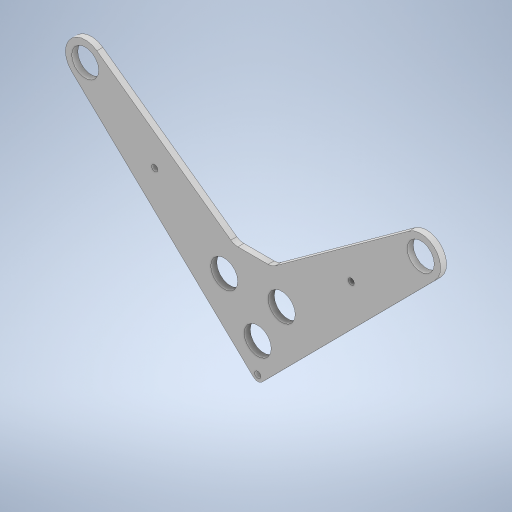
# Autodesk Inventor part: MainBody
Saved by Autodesk Inventor 2024.3 (Build 283343000, 343)
## iProperties
Created: 2024-09-01
Part Number: MainBody
Material: Generic
Document SubType Name: Modeling
Designer: isaac
Density: 1 g/cm^3
Appearance: Default
Author: isaac
Autodesk Inventor part; units mm, degrees
ref_plane "YZ Plane" through (0, 0, 0) normal (1, 0, 0) x (0, 1, 0)
ref_plane "XZ Plane" through (0, 0, 0) normal (0, 1, 0) x (-1, 0, 0)
ref_plane "XY Plane" through (0, 0, 0) normal (0, 0, 1) x (1, 0, 0)
sketch "Sketch1" plane through (0, 0, 0) normal (0, 0, 1) x (1, 0, 0)
  circle A0 centre (0, 0) radius 20.32 construction
  circle A1 centre (25.4496, 43.9654) radius 30.48 construction
  circle A2 centre (-35.5104, 43.9654) radius 30.48 construction
  circle A3 centre (-35.5104, 43.9654) radius 31.75 construction
  circle A4 centre (0, 0) radius 21.59 construction
  line L0 (-15.5607, 19.2657) -> (-13.5658, 16.7958) construction
  circle A5 centre (25.4496, 43.9654) radius 31.75 construction
  circle A6 centre (-35.5104, 43.9654) radius 14.351
  circle A7 centre (0, 0) radius 14.351
  circle A8 centre (25.4496, 43.9654) radius 14.351
  line L1 (25.4496, 43.9654) -> (172.7696, 163.9395) construction
  line L2 (-35.5104, 43.9654) -> (-182.8304, 163.9395) construction
  circle A9 centre (172.7696, 163.9395) radius 50.8 construction
  circle A10 centre (-182.8304, 163.9395) radius 50.8 construction
  line L3 (-132.0304, 163.9395) -> (121.9696, 163.9395) construction
  circle A11 centre (-182.8304, 163.9395) radius 14.351
  circle A12 centre (172.7696, 163.9395) radius 14.351
  circle A13 centre (0, -31.115) radius 6.35 construction
  line L4 (0, -21.59) -> (0, -24.765) construction
  circle A14 centre (-109.1704, 103.9524) radius 6.35 construction
  circle A15 centre (99.1096, 103.9524) radius 6.35 construction
  circle A16 centre (-109.1704, 103.9524) radius 3.2639
  circle A17 centre (99.1096, 103.9524) radius 3.2639
  circle A18 centre (0, -31.115) radius 3.2639
  line L5 (-21.1034, 75.7154) -> (11.0426, 75.7154)
  circle A19 centre (172.7696, 163.9395) radius 21.0058 construction
  circle A20 centre (-182.8304, 163.9395) radius 21.0058 construction
  line L6 (-170.5082, 180.9515) -> (-28.5533, 78.1301)
  line L7 (18.4926, 78.1301) -> (160.4474, 180.9515)
  line L8 (187.6857, 149.1492) -> (4.5091, -35.5861)
  line L9 (-4.3879, -35.7051) -> (-197.3457, 148.7556)
  arc A21 (-4.3879, -35.7051) -> (4.5091, -35.5861) centre (0, -31.115) ccw
  arc A22 (-170.5082, 180.9515) -> (-197.3457, 148.7556) centre (-182.8304, 163.9395) ccw
  arc A23 (187.6857, 149.1492) -> (160.4474, 180.9515) centre (172.7696, 163.9395) ccw
  arc A24 (11.0426, 75.7154) -> (18.4926, 78.1301) centre (11.0426, 88.4154) ccw
  arc A25 (-28.5533, 78.1301) -> (-21.1034, 75.7154) centre (-21.1034, 88.4154) ccw
  point P0 (-17.1517, 69.8695)
  point P1 (15.1589, 75.7154)
  point P2 (15.3395, 75.7154)
  point P3 (184.7885, 149.1595)
  point P4 (-25.2197, 75.7154)
  dimension "d7" = 101.6
  dimension "d0" = 40.64
  dimension "d1" = 60.96
  dimension "d2" = 63.5
  dimension "d3" = 43.18
  dimension "d4" = 3.175
  dimension "d5" = 28.702
  dimension "d6" = 189.992
  dimension "d8" = 254
  dimension "d9" = 28.702
  dimension "d10" = 12.7
  dimension "d11" = 3.175
  dimension "d12" = 12.7
  dimension "d13" = 12.7
  dimension "d14" = 6.5278
  dimension "d15" = 6.5278
  dimension "d16" = 42.0116
  dimension "d21" = 12.7
  dimension "d22" = 12.7
  constraints: 24 centre point, 20 end point, 20 point on circle, 20 tangent, 16 coincident, 9 equal radius, 9 point on line, 4 horizontal alignment, 2 midpoint, 1 equal length, 1 horizontal, 1 vertical, 4 other
  measures "d0" diameter of A0
  measures "d1" diameter of A1
  measures "d2" diameter of A3
  measures "d3" diameter of A4
  measures "d4" distance of L0.start L0.end
  measures "d5" diameter of A8
  measures "d6" distance of L1.start L1.end
  measures "d8" distance of L3.start L3.end
  measures "d9" diameter of A11
  measures "d10" diameter of A13
  measures "d11" distance of L4.start L4.end
  measures "d12" diameter of A14
  measures "d13" diameter of A15
  measures "d14" diameter of A16
  measures "d15" diameter of A17
  measures "d16" diameter of A19
  measures "d21" radius of A24
  measures "d22" radius of A25
extrude "Extrusion2" add sketch "Sketch1" along normal blind 6.35
body "Solid2"
